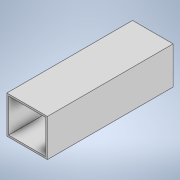
# Autodesk Inventor part: bido
Saved by Autodesk Inventor 2020.2 (Build 242310000, 310)
## iProperties
Created: 2020-03-27
Part Number: bido
Material: Generic
Document SubType Name: Modeling
Designer: iamin
Density: 1 g/cm^3
Appearance: Default
Author: iamin
Autodesk Inventor part; units mm, degrees
ref_plane "YZ Plane" through (0, 0, 0) normal (1, 0, 0) x (0, 1, 0)
ref_plane "XZ Plane" through (0, 0, 0) normal (0, 1, 0) x (-1, 0, 0)
ref_plane "XY Plane" through (0, 0, 0) normal (0, 0, 1) x (1, 0, 0)
sketch "Sketch1" plane through (0, 0, 0) normal (0, 0, 1) x (1, 0, 0)
  line L0 (0, 0) -> (42, 0)
  line L1 (42, 0) -> (42, 38.66)
  line L2 (42, 38.66) -> (0, 38.66)
  line L3 (0, 38.66) -> (0, 0)
  line L4 (40.2, 1.8) -> (1.8, 1.8)
  line L5 (1.8, 1.8) -> (1.8, 36.86)
  line L6 (1.8, 36.86) -> (40.2, 36.86)
  line L7 (40.2, 36.86) -> (40.2, 1.8)
  dimension "d0" = 42
  dimension "d1" = 38.66
  dimension "d2" = 1.8
  constraints: 16 end point, 4 parallel, 2 perpendicular, 1 horizontal, 3 other
  measures "d0" distance of L2.end L1.end
  measures "d1" distance between parallel lines of L0 L2
  measures "d2" distance between parallel lines of L0 L4
extrude "Extrusion1" add sketch "Sketch1" along normal mid plane 130
body "Solid1"
